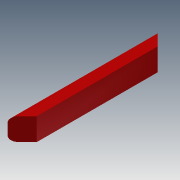
# Autodesk Inventor part: bumper front
Saved by Autodesk Inventor 2014 (Build 180170000, 170)
## iProperties
Created: 2016-01-12
Part Number: bumper front
Material: Wood (Birch)
Document SubType Name: Modeling
Designer: Paul
Density: 0.55 g/cm^3
Appearance: Red
Mass: 4231.29 g
Surface Area: 3269.68 cm^2
Volume: 7693.25 cm^3
Author: Paul
Autodesk Inventor part; units mm, degrees
ref_plane "YZ Plane" through (0, 0, 0) normal (1, 0, 0) x (0, 1, 0)
ref_plane "XZ Plane" through (0, 0, 0) normal (0, 1, 0) x (-1, 0, 0)
ref_plane "XY Plane" through (0, 0, 0) normal (0, 0, 1) x (1, 0, 0)
sketch "Sketch1" plane through (0, 0, 0) normal (0, 0, 1) x (1, 0, 0)
  line L0 (0, 0) -> (19.05, 0)
  line L1 (19.05, 0) -> (19.05, 127)
  line L2 (19.05, 127) -> (0, 127)
  line L3 (0, 127) -> (0, 0)
  circle A0 centre (-31.75, 95.25) radius 31.75
  circle A1 centre (-31.75, 31.75) radius 31.75
  line L4 (0, 127) -> (-31.75, 127)
  line L5 (0, 0) -> (-31.75, 0)
  line L6 (-63.5, 31.75) -> (-63.5, 95.25)
  dimension "d0" = 19.05
  dimension "d1" = 127
  dimension "d2" = 63.5
  dimension "d3" = 63.5
  dimension "d4" = 31.75
  constraints: 14 end point, 7 tangent, 4 point on circle, 2 centre point, 2 parallel, 1 horizontal, 1 perpendicular
  measures "d0" distance of L2.end L1.end
  measures "d1" distance of L1.end L0.end
  measures "d2" diameter of A0
  measures "d3" diameter of A1
  measures "d4" distance from line of A1.centre L0
extrude "Extrusion1" add sketch "Sketch1" along normal blind 850.9
sketch "Sketch2" plane through (-31.75, 127, 0) normal (0, 1, 0) x (1, 0, 0)
  line L0 (50.8, 0) -> (50.8, -850.9) projected
  line L1 (-31.75, 0) -> (-31.75, -850.9) projected
  line L2 (-31.75, 0) -> (50.8, -82.55)
  line L3 (-31.75, 0) -> (95.25, 0) construction
  line L4 (-31.75, 0) -> (50.8, 0)
  line L5 (50.8, 0) -> (50.8, -82.55)
  line L6 (-31.75, -850.9) -> (50.8, -768.35)
  line L7 (-31.75, -850.9) -> (95.25, -850.9) construction
  line L8 (-31.75, -850.9) -> (50.8, -850.9)
  line L9 (50.8, -850.9) -> (50.8, -768.35)
  point P0 (31.75, 0)
  dimension "d8" = 45
  dimension "d10" = 45
  constraints: 16 end point, 2 collinear, 2 horizontal, 2 point on line, 1 perpendicular
  measures "d8" angle of L2 L3
  measures "d10" angle of L7 L6
extrude "Extrusion2" cut sketch "Sketch2" against normal blind 127 contours L0 L2 L4 | L0 L8 L6
body "Solid1"
